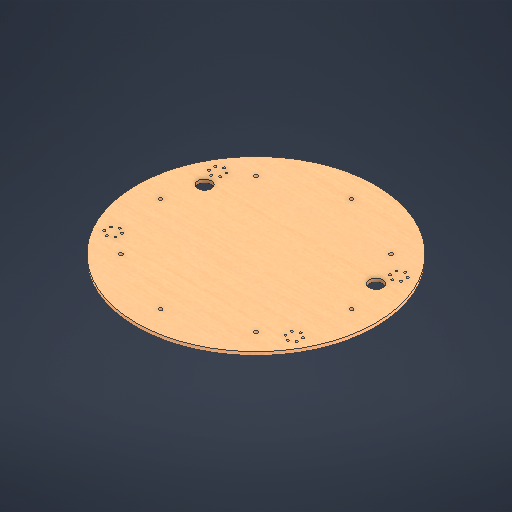
# Autodesk Inventor part: layer5_new
Saved by Autodesk Inventor 2026 (Build 300175050, 175E)
## iProperties
Created: 2025-06-05
Part Number: layer5_new
Material: Generic
Document SubType Name: Modeling
Designer: satom
Density: 1 g/cm^3
Appearance: Default
Author: satom
Autodesk Inventor part; units mm, degrees
ref_plane "YZ Plane" through (0, 0, 0) normal (1, 0, 0) x (0, 1, 0)
ref_plane "XZ Plane" through (0, 0, 0) normal (0, 1, 0) x (-1, 0, 0)
ref_plane "XY Plane" through (0, 0, 0) normal (0, 0, 1) x (1, 0, 0)
sketch "Sketch1" plane through (0, 0, 0) normal (0, 1, 0) x (-1, 0, 0)
  circle A0 centre (0, 0) radius 177
  dimension "d0" = 354
  constraints: 1 centre point, 1 coincident
  measures "d0" diameter of A0
extrude "Extrusion1" add sketch "Sketch1" along normal blind 5
sketch "Sketch2" plane through (0, 5, 0) normal (0, 1, 0) x (1, 0, 0)
  line L0 (0, 0) -> (153.2865, -88.5) construction
  circle A0 centre (0, 0) radius 177 construction
  line L1 (-177, 0) -> (177, 0) construction
  circle A1 centre (142.288, -82.15) radius 1.7
  line L2 (142.288, -82.15) -> (134.0391, -77.3875) construction
  circle A2 centre (142.288, -72.625) radius 1.7
  circle A3 centre (134.0391, -67.8625) radius 1.7
  circle A4 centre (125.7902, -72.625) radius 1.7
  circle A5 centre (125.7902, -82.15) radius 1.7
  circle A6 centre (134.0391, -86.9125) radius 1.7
  circle A7 centre (142.288, 82.15) radius 1.7
  circle A8 centre (142.288, 72.625) radius 1.7
  circle A9 centre (134.0391, 67.8625) radius 1.7
  circle A10 centre (125.7902, 72.625) radius 1.7
  circle A11 centre (125.7902, 82.15) radius 1.7
  circle A12 centre (134.0391, 86.9125) radius 1.7
  line L3 (0, 177) -> (0, -177) construction
  circle A13 centre (0, 0) radius 177 construction
  circle A14 centre (-142.288, -82.15) radius 1.7
  circle A15 centre (-142.288, -72.625) radius 1.7
  circle A16 centre (-134.0391, -67.8625) radius 1.7
  circle A17 centre (-125.7902, -72.625) radius 1.7
  circle A18 centre (-125.7902, -82.15) radius 1.7
  circle A19 centre (-134.0391, -86.9125) radius 1.7
  circle A20 centre (-134.0391, 67.8625) radius 1.7
  circle A21 centre (-142.288, 72.625) radius 1.7
  circle A22 centre (-142.288, 82.15) radius 1.7
  circle A23 centre (-134.0391, 86.9125) radius 1.7
  circle A24 centre (-125.7902, 82.15) radius 1.7
  circle A25 centre (-125.7902, 72.625) radius 1.7
  dimension "d3" = 30
  dimension "d4" = 3.4
  dimension "d5" = 12.7
  dimension "d6" = 9.525
  dimension "d9" = 360
  constraints: 25 centre point, 18 symmetric about line, 8 end point, 5 point on circle, 2 point on line, 1 horizontal, 1 perpendicular, 32 other
  measures "d3" angle of L1 L0
  measures "d4" diameter of A1
  measures "d5" distance of L0.end L2.start
  measures "d6" distance of L2.start L2.end
extrude "Standoffs" cut sketch "Sketch2" against normal through all
sketch "Sketch3" plane through (0, 5, 0) normal (0, 1, 0) x (1, 0, 0)
  circle A0 centre (-127, 50.8) radius 10.16
  circle A1 centre (127, 50.8) radius 10.16
  circle A2 centre (0, 0) radius 177 construction
  circle A3 centre (0, 0) radius 177 construction
  line L0 (0, 0) -> (0, 177) construction
  line L1 (0, 0) -> (177, 0) construction
  line L2 (0, 0) -> (-177, 0) construction
  dimension "d13" = 20.32
  dimension "d14" = 20.32
  dimension "d19" = 127
  dimension "d20" = 127
  dimension "d21" = 50.8
  dimension "d22" = 50.8
  constraints: 6 end point, 3 point on circle, 2 centre point, 1 horizontal, 1 point on line, 1 vertical
  measures "d13" diameter of A0
  measures "d14" diameter of A1
  measures "d19" distance from line of L0 A0.centre
  measures "d20" distance from line of L0 A1.centre
  measures "d21" distance from line of L2 A0.centre
  measures "d22" distance from line of L1 A1.centre
extrude "Wires" cut sketch "Sketch3" against normal through all
sketch "Sketch4" plane through (0, 5, 0) normal (0, 1, 0) x (1, 0, 0)
  circle A0 centre (0, -141.44) radius 2.667
  circle A1 centre (0, 0) radius 177 construction
  line L0 (0, 0) -> (0, -177) construction
  line L1 (0, -177) -> (48.7641, -177) construction
  circle A2 centre (100.0132, -100.0132) radius 2.667
  circle A3 centre (141.44, 0) radius 2.667
  circle A4 centre (100.0132, 100.0132) radius 2.667
  circle A5 centre (0, 141.44) radius 2.667
  circle A6 centre (-100.0132, 100.0132) radius 2.667
  circle A7 centre (-141.44, 0) radius 2.667
  circle A8 centre (-100.0132, -100.0132) radius 2.667
  dimension "d25" = 5.334
  dimension "d28" = 35.56
  dimension "d31" = 360
  constraints: 8 centre point, 4 end point, 1 horizontal, 1 point on line, 1 vertical, 1 vertical alignment, 18 other
  measures "d25" diameter of A0
  measures "d28" distance from line of L1 A0.centre
extrude "Zip Ties" cut sketch "Sketch4" against normal through all
equation "\"d0\" = robot_diameter"
equation "\"d1\" = hardboard_thickness"
equation "\"d4\" = m3_clearance"
equation "\"d14\" = d13"
equation "\"d22\" = d21"
equation "\"m3_heat_set_insert\" = 4"
equation "\"m3_clearance\" = 3.4"
equation "\"m3_heat_set_depth\" = 7"
equation "\"robot_diameter\" = 354"
equation "\"hardboard_thickness\" = 5"
body "Solid1"
